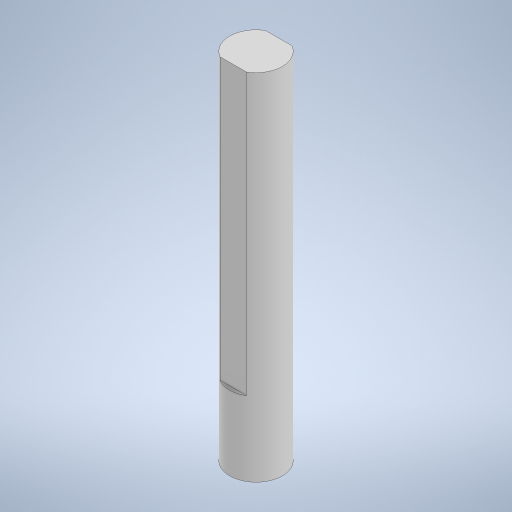
# Autodesk Inventor part: Stang
Saved by Autodesk Inventor 2023 (Build 270158000, 158)
## iProperties
Created: 2023-03-15
Part Number: Stang
Material: Generic
Document SubType Name: Modeling
Designer: daanj
Density: 1 g/cm^3
Appearance: Default
Author: daanj
Autodesk Inventor part; units mm, degrees
ref_plane "YZ Plane" through (0, 0, 0) normal (1, 0, 0) x (0, 1, 0)
ref_plane "XZ Plane" through (0, 0, 0) normal (0, 1, 0) x (-1, 0, 0)
ref_plane "XY Plane" through (0, 0, 0) normal (0, 0, 1) x (1, 0, 0)
sketch "Sketch1" plane through (0, 0, 0) normal (0, 1, 0) x (-1, 0, 0)
  circle A0 centre (0, 0) radius 3
  dimension "d0" = 6
  constraints: 1 centre point, 1 coincident
  measures "d0" diameter of A0
extrude "Extrusion1" add sketch "Sketch1" along normal blind 8.5
sketch "Sketch2" plane through (0, 8.5, 0) normal (0, 1, 0) x (1, 0, 0)
  circle A0 centre (0, 0) radius 3 projected
  circle A1 centre (0, 0) radius 3 projected
  line L0 (-1.5, 2.5981) -> (1.5, 2.5981)
  line L1 (-1.5, -2.5981) -> (1.5, -2.5981)
  arc A2 (-1.5, 2.5981) -> (-1.5, -2.5981) centre (0, 0) ccw
  arc A3 (1.5, -2.5981) -> (1.5, 2.5981) centre (0, 0) ccw
  point P0 (1.5, -2.5981)
  dimension "d3" = 3
  constraints: 6 point on circle, 4 end point, 2 centre point, 2 horizontal, 1 coincident
  measures "d3" distance of L0.start L0.end
extrude "Extrusion2" add sketch "Sketch2" along normal blind 32 contours A0 L1 L0
body "Solid1"
